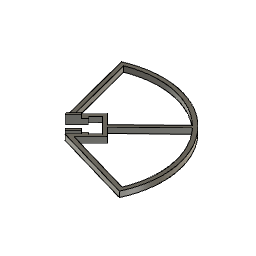
Prop_guard_clamp v2 (Autodesk Fusion 360 design; units mm, degrees)
Autodesk Fusion 360 part; units mm, degrees
sketch "Sketch1" plane through (0, 0, 0) normal (0, 0, 1) x (1, 0, 0)
  line L0 (41.26, -53.9475) -> (-23.8891, -34.972)
  arc A0 (41.26, -53.9475) -> (-52.9571, 42.103) centre (-23.9263, -23.6549) ccw
  line L1 (-49.1844, 40.1007) -> (-34.6167, -16.2167)
  line L2 (-34.6167, -16.2167) -> (-20.6815, -2.1702)
  line L3 (-3.8871, -18.8317) -> (-18.0593, -33.1169)
  line L4 (-18.0593, -33.1169) -> (39.4437, -49.8653)
  arc A1 (23.8726, 25.5184) -> (-49.1844, 40.1007) centre (-23.9263, -23.6549) ccw
  line L5 (23.8726, 25.5184) -> (-12.7212, -10.0675)
  line L6 (25.8056, 23.5625) -> (-10.9878, -11.7872)
  arc A2 (39.4437, -49.8653) -> (25.8056, 23.5625) centre (-23.9263, -23.6549) ccw
  line L7 (23.8726, 25.5184) -> (28.5034, 25.5184) construction
  line L8 (-20.6815, -2.1702) -> (-12.7212, -10.0675)
  line L9 (-10.9878, -11.7872) -> (-3.8871, -18.8317)
  line L10 (-36.4169, -21.8399) -> (-29.7834, -15.1535)
  line L11 (-20.9093, -6.2086) -> (-8.0298, -18.9862)
  line L12 (-16.9038, -27.9311) -> (-23.8891, -34.972)
  line L13 (-52.9571, 42.103) -> (-36.4169, -21.8399)
  line L14 (-8.0298, -18.9862) -> (-14.0867, -25.0914)
  line L15 (-14.0867, -25.0914) -> (-15.5065, -23.6828)
  line L16 (-15.5065, -23.6828) -> (-18.3237, -26.5225)
  line L17 (-18.3237, -26.5225) -> (-16.9038, -27.9311)
  line L18 (-26.9662, -12.3138) -> (-20.9093, -6.2086)
  line L19 (-26.9662, -12.3138) -> (-25.5464, -13.7224)
  line L20 (-25.5464, -13.7224) -> (-28.3636, -16.562)
  line L21 (-28.3636, -16.562) -> (-29.7834, -15.1535)
  line L22 (-18.3237, -26.5225) -> (-25.3088, -33.5634)
  line L23 (-25.3088, -33.5634) -> (-23.8891, -34.972)
  line L24 (-36.4169, -21.8399) -> (-34.9971, -23.2485)
  line L25 (-34.9971, -23.2485) -> (-28.3636, -16.562)
  dimension "d4" = 2
  dimension "d5" = 4
  dimension "d6" = 2
  dimension "d7" = 4
  dimension "d8" = 9.918
  dimension "d9" = 2
  constraint perpendicular L2 L8
  constraint perpendicular L3 L8
  constraint parallel L0 L4
  constraint concentric A0 A1
  constraint coincident L6.end L8
  constraint concentric A1 A2
  constraint coincident A0 L7.end
  constraint horizontal L7
  constraint parallel L2 L10
  constraint perpendicular L10 L11
  constraint parallel L1 L13
  constraint parallel L3 L12
  constraint parallel L3 L14
  constraint perpendicular L14 L15
  constraint perpendicular L15 L16
  constraint perpendicular L12 L17
  constraint parallel L2 L18
  constraint perpendicular L10 L19
  constraint perpendicular L19 L20
  constraint perpendicular L10 L21
  constraint perpendicular L17 L22
  constraint perpendicular L10 L24
  measures "d4" distance of L14.end L15.end
  measures "d5" distance of L15.end L16.end
  measures "d6" distance of L18.start L19.end
  measures "d7" distance of L19.end L20.end
  measures "d8" distance of L16.end L22.end
  measures "d9" distance of L10.start L24.end
extrude "Extrude1" add sketch "Sketch1" along normal blind 4.7
sketch "Sketch2" plane through (0, 0, 4.7) normal (0, 0, 1) x (-1, 0, 0)
  arc A0 (-23.8726, -25.5184) -> (49.1844, -40.1007) centre (23.9263, 23.6549) ccw
  line L0 (-23.8726, -25.5184) -> (12.7212, 10.0675)
  line L1 (12.7212, 10.0675) -> (20.6815, 2.1702)
  line L2 (20.6815, 2.1702) -> (34.6167, 16.2167)
  line L3 (34.6167, 16.2167) -> (49.1844, -40.1007)
  line L4 (3.8871, 18.8317) -> (10.9878, 11.7872)
  line L5 (10.9878, 11.7872) -> (-25.8056, -23.5625)
  arc A1 (-39.4437, 49.8653) -> (-25.8056, -23.5625) centre (23.9263, 23.6549) ccw
  line L6 (-39.4437, 49.8653) -> (18.0593, 33.1169)
  line L7 (18.0593, 33.1169) -> (3.8871, 18.8317)
  arc A2 (-41.26, 53.9475) -> (52.9571, -42.103) centre (23.9263, 23.6549) ccw
  line L8 (52.9571, -42.103) -> (36.4169, 21.8399)
  line L9 (36.4169, 21.8399) -> (34.9971, 23.2485)
  line L10 (34.9971, 23.2485) -> (25.5464, 13.7224)
  line L11 (25.5464, 13.7224) -> (26.9662, 12.3138)
  line L12 (26.9662, 12.3138) -> (20.9093, 6.2086)
  line L13 (20.9093, 6.2086) -> (8.0298, 18.9862)
  line L14 (8.0298, 18.9862) -> (14.0867, 25.0914)
  line L15 (14.0867, 25.0914) -> (15.5065, 23.6828)
  line L16 (15.5065, 23.6828) -> (25.3088, 33.5634)
  line L17 (25.3088, 33.5634) -> (23.8891, 34.972)
  line L18 (23.8891, 34.972) -> (-41.26, 53.9475)
  line L19 (16.9038, 27.9311) -> (18.3237, 26.5225)
  line L20 (16.9038, 27.9311) -> (23.8891, 34.972)
  line L21 (36.4169, 21.8399) -> (29.7834, 15.1535)
  line L22 (29.7834, 15.1535) -> (28.3636, 16.562)
  dimension "d12" = 4
  dimension "d13" = 4
  constraint coincident L17.end L18.start
  constraint coincident L16 L19.end
  constraint perpendicular L16 L19
  constraint coincident L8.end L9.start
  constraint coincident L10 L22.end
  constraint perpendicular L10 L22
  measures "d12" distance of L14.end L19.start
  measures "d13" distance of L11.end L21.end
extrude "Extrude2" add sketch "Sketch2" along normal blind 2.8 contours L16 L17 L19 L20 | L9 L10 L21 L22
